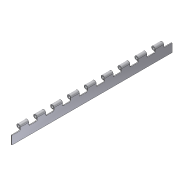
# Autodesk Inventor part: FE-00004-03B
Saved by Autodesk Inventor 2012 (Build 160160000, 160)
## iProperties
Created: 2008-05-29
Part Number: FE-00004-03B
Document SubType Name: Modeling
Designer: narosenberg
Density: 1 g/cm^3
Mass: 44.4373 g
Surface Area: 424.606 cm^2
Volume: 44.4373 cm^3
Material: Default
Author: narosenberg
Autodesk Inventor part; units mm, degrees
ref_plane "YZ Plane" through (0, 0, 0) normal (1, 0, 0) x (0, 1, 0)
ref_plane "XZ Plane" through (0, 0, 0) normal (0, 1, 0) x (-1, 0, 0)
ref_plane "XY Plane" through (0, 0, 0) normal (0, 0, 1) x (1, 0, 0)
sketch "Sketch1" plane through (0, 0, 0) normal (0, 0, 1) x (1, 0, 0)
  line L0 (-3.3994, 19.4704) -> (-3.3994, -14.4081)
  line L1 (-3.3994, -14.4081) -> (-5.6854, -14.4081)
  arc A0 (-3.3994, 19.4704) -> (-6.6643, 14.3475) centre (-9.0509, 19.4704) ccw
  arc A1 (-5.6854, 19.4704) -> (-7.7383, 16.3714) centre (-9.0509, 19.4704) ccw
  line L2 (-7.7383, 16.3714) -> (-6.6643, 14.3475)
  line L3 (-5.6854, -14.4081) -> (-5.6854, 19.4704)
  dimension "d0" = 11.303
  dimension "d2" = 2.286
  constraints: 8 end point, 4 point on circle, 2 centre point, 2 tangent, 1 coincident, 1 parallel
  measures "d0" diameter of A0
  measures "d2" distance between parallel lines of L0 L3
extrude "Extrusion1" add sketch "Sketch1" along normal blind 482.6
sketch "Sketch2" plane through (-3.3994, -14.4081, 0) normal (1, 0, 0) x (0, 0, -1)
  line L0 (-482.6, 50.4757) -> (-457.2, 50.4757)
  line L1 (-457.2, 50.4757) -> (-457.2, 25.052)
  line L2 (-457.2, 25.052) -> (-482.6, 25.052)
  line L3 (-482.6, 25.052) -> (-482.6, 50.4757)
  line L4 (-482.6, 37.244) -> (0, 37.244) projected
  line L5 (-482.6, 33.8785) -> (-482.6, 30.7795) projected
  line L6 (0, 30.7795) -> (-482.6, 30.7795) projected
  line L7 (0, 30.7795) -> (0, 33.8785) projected
  line L8 (0, 33.8785) -> (-482.6, 33.8785) projected
  line L9 (0, 28.227) -> (-482.6, 28.227) projected
  dimension "d6" = 25.4
  dimension "d7" = 3.175
  constraints: 8 end point, 2 parallel, 1 horizontal, 1 perpendicular
  measures "d6" distance of L0.start L0.end
  measures "d7" distance between parallel lines of L2 L9
extrude "Extrusion2" cut sketch "Sketch2" against normal through all contours L0 L1 L4 L3 | L4 L1 L8 L3 | L8 L1 L6 L3 | L6 L1 L9 L3 | L9 L1 L2 L3
pattern_linear "Rectangular Pattern1" count 10 spacing 50.8 along (0, 0, -1) of "Extrusion2"
fillet "Fillet2" radius 3.175 18 edges at (-4.5424, 10.6439, 381) (-4.5424, 10.6439, 355.6) (-4.5424, 10.6439, 330.2) (-4.5424, 10.6439, 304.8) (-4.5424, 10.6439, 279.4) (-4.5424, 10.6439, 254) (-4.5424, 10.6439, 228.6) (-4.5424, 10.6439, 203.2) (-4.5424, 10.6439, 177.8) (-4.5424, 10.6439, 152.4) (-4.5424, 10.6439, 127) (-4.5424, 10.6439, 101.6) (-4.5424, 10.6439, 76.2) (-4.5424, 10.6439, 50.8) (-4.5424, 10.6439, 25.4) (-4.5424, 10.6439, 431.8) (-4.5424, 10.6439, 406.4) (-4.5424, 10.6439, 457.2)
body "Solid1"
